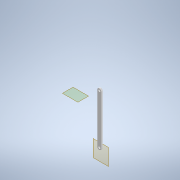
# Autodesk Inventor part: horizontal bottom trusses
Saved by Autodesk Inventor 2020 (Build 240168000, 168)
## iProperties
Created: 2020-07-05
Part Number: horizontal bottom trusses
Material: Generic
Document SubType Name: Modeling
Designer: Ashiqrahman
Density: 1 g/cm^3
Appearance: Default
Author: Ashiqrahman
Autodesk Inventor part; units mm, degrees
ref_plane "YZ Plane" through (0, 0, 0) normal (1, 0, 0) x (0, 1, 0)
ref_plane "XZ Plane" through (0, 0, 0) normal (0, 1, 0) x (-1, 0, 0)
ref_plane "XY Plane" through (0, 0, 0) normal (0, 0, 1) x (1, 0, 0)
ref_plane "Work Plane1" through (0, -25.5202, -99.7789) normal (0, -1, 0) x (-1, 0, 0)
ref_plane "Work Plane2" through (150, 0, 0) normal (0, 0, 1) x (1, 0, 0)
sketch "Sketch1" plane through (150, 0, 0) normal (0, 0, 1) x (1, 0, 0)
  line L0 (-4.7216, 11.5478) -> (-13.9385, -14.9025) projected
  line L1 (-13.9385, -14.9025) -> (13.9385, -14.9025) projected
  line L2 (13.9385, -14.9025) -> (4.7216, 11.5478) projected
  arc A0 (4.7216, 11.5478) -> (-4.7216, 11.5478) centre (0, 9.9025) ccw projected
  line L3 (-4.7216, 11.5478) -> (-13.9385, -14.9025) projected
  circle A1 centre (0, 9.9025) radius 2 projected
  arc A2 (-4.7216, 106.1118) -> (4.7216, 106.1118) centre (0, 107.7571) ccw projected
  line L4 (4.7216, 106.1118) -> (13.9385, 132.5621) projected
  line L5 (13.9385, 132.5621) -> (-13.9385, 132.5621) projected
  line L6 (-13.9385, 132.5621) -> (-4.7216, 106.1118) projected
  circle A3 centre (0, 107.7571) radius 2 projected
  line L7 (0, 9.9025) -> (0, 107.7571) construction
  line L8 (4, 9.9025) -> (4, 107.7571)
  line L9 (-4, 107.7571) -> (-4, 9.9025)
  arc A4 (-4, 9.9025) -> (4, 9.9025) centre (0, 9.9025) ccw
  arc A5 (4, 107.7571) -> (-4, 107.7571) centre (0, 107.7571) ccw
  point P0 (-150, 0)
  point P1 (0, 58.8298)
  dimension "d0" = 8
  constraints: 8 end point, 4 point on circle, 4 tangent, 2 centre point, 1 midpoint, 1 parallel
  measures "d0" diameter of A5
extrude "Extrusion1" add sketch "Sketch1" along normal blind 3 contours L9 A2 L8 A0 | A0 L8 A4 L9 | L9 A5 L8 A2
body "Solid1"
